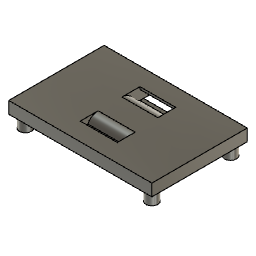
ObudowaOkienko v1 (Autodesk Fusion 360 design; units mm, degrees)
Autodesk Fusion 360 part; units mm, degrees
sketch "Sketch1" plane through (0, 0, 0) normal (0, 0, 1) x (1, 0, 0)
  line L0 (-100, 75) -> (20, 75)
  line L1 (20, 75) -> (20, -5)
  line L2 (20, -5) -> (-100, -5)
  line L3 (-100, -5) -> (-100, 75)
  constraint horizontal L0
  constraint vertical L1
  constraint horizontal L2
  constraint vertical L3
extrude "Extrude1" add sketch "Sketch1" along normal blind 10
sketch "Sketch2" plane through (0, 0, 10) normal (0, 0, 1) x (-1, 0, 0)
  line L0 (100, 5) -> (-20, 5)
  line L1 (-20, 5) -> (-20, -75)
  line L2 (-20, -75) -> (100, -75)
  line L3 (100, -75) -> (100, 5)
  circle A0 centre (93, -68) radius 5
  circle A1 centre (-13, -68) radius 5
  circle A2 centre (-13, -2) radius 5
  circle A3 centre (93, -2) radius 5
  line L4 (88, -63) -> (-8, -63)
  line L5 (-8, -63) -> (-8, -7)
  line L6 (-8, -7) -> (88, -7)
  line L7 (88, -7) -> (88, -63)
  dimension "d3" = 10
  constraint horizontal L4
  constraint vertical L5
  constraint horizontal L6
  constraint vertical L7
  measures "d3" diameter of A3
extrude "Extrude2" add sketch "Sketch2" along normal blind 10 contours A0 | A1 | A2 | A3 | L4 L5 L6 L7
move_body "Move1" bodies 1 to x (-1, 0, 0) y (0, 1, 0) z (0, 0, -1) at (16, 0, 40)
move_body "Move2" bodies 1 to x (1, 0, 0) y (0, 1, 0) z (0, 0, 1) at (-1, 0, 0)
move_body "Move3" bodies 1 to x (1, 0, 0) y (0, 1, 0) z (0, 0, 1) at (0, 0, -20)
sketch "Sketch3" plane through (0, 0, 20) normal (0, 0, 1) x (-1, 0, 0)
  line L0 (5, 5) -> (-115, 5)
  line L1 (-115, 5) -> (-115, -75)
  line L2 (-115, -75) -> (5, -75)
  line L3 (5, -75) -> (5, 5)
  line L4 (-40, -60) -> (-70, -60)
  line L5 (-70, -60) -> (-70, -55)
  line L6 (-70, -55) -> (-40, -55)
  line L7 (-40, -55) -> (-40, -60)
  line L8 (-40, -15) -> (-71, -15)
  line L9 (-71, -15) -> (-71, -10)
  line L10 (-71, -10) -> (-40, -10)
  line L11 (-40, -10) -> (-40, -15)
  constraint horizontal L4
  constraint vertical L5
  constraint horizontal L6
  constraint vertical L7
  constraint horizontal L8
  constraint vertical L9
  constraint horizontal L10
  constraint vertical L11
extrude "Extrude3" cut sketch "Sketch3" against normal blind 10 contours L4 L5 L6 L7 | L8 L9 L10 L11
fillet "Fillet1" radius 10 1 faces at (50.3333, 15, 16.6667)
fillet "Fillet2" radius 10 1 faces at (60, 55, 16.6667)
sketch "Sketch4" plane through (0, 10, 0) normal (0, 1, 0) x (-1, 0, 0)
  line L0 (-40, 20) -> (-71, 20)
  line L1 (-71, 20) -> (-71, 10)
  line L2 (-71, 10) -> (-40, 10)
  line L3 (-40, 10) -> (-40, 20)
  line L4 (-71, 18) -> (-40, 18)
  line L5 (-40, 18) -> (-40, 10)
  line L6 (-40, 10) -> (-71, 10)
  line L7 (-71, 10) -> (-71, 18)
  constraint horizontal L4
  constraint vertical L5
  constraint horizontal L6
  constraint vertical L7
  constraint coincident L2.end L3.start
  constraint coincident L1 L4.start
extrude "Extrude4" cut sketch "Sketch4" against normal blind 8 contours L1 L2 L3 L4 L5 L6 L7
sketch "Sketch5" plane through (0, 60, 0) normal (0, -1, 0) x (1, 0, 0)
  line L0 (70, 20) -> (40, 20)
  line L1 (40, 20) -> (40, 10)
  line L2 (40, 10) -> (70, 10)
  line L3 (70, 10) -> (70, 20)
  line L4 (40, 18) -> (70, 18)
  line L5 (70, 18) -> (70, 10)
  line L6 (70, 10) -> (40, 10)
  line L7 (40, 10) -> (40, 18)
  constraint horizontal L4
  constraint vertical L5
  constraint horizontal L6
  constraint vertical L7
  constraint coincident L2.end L3.start
  constraint coincident L1 L4.start
extrude "Extrude5" cut sketch "Sketch5" against normal blind 8 contours L1 L2 L3 L4 L5 L6 L7
